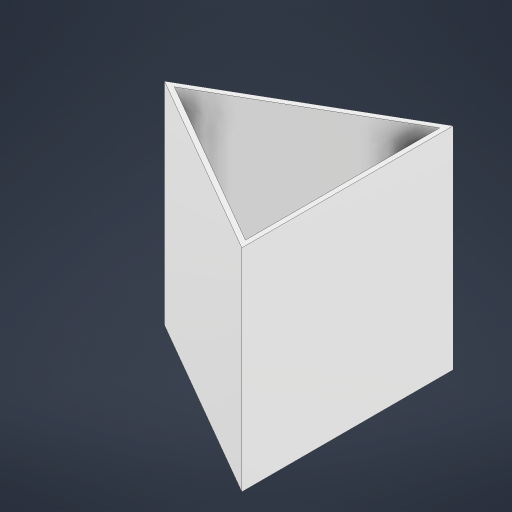
# Autodesk Inventor part: Triangle
Saved by Autodesk Inventor 2023 (Build 270158000, 158)
## iProperties
Created: 2023-11-15
Part Number: Triangle
Material: ABS Plastic
Document SubType Name: Modeling
Designer: dexter.hedman
Density: 1.06 g/cm^3
Appearance: Smooth - White
Author: dexter.hedman
Autodesk Inventor part; units mm, degrees
ref_plane "YZ Plane" through (0, 0, 0) normal (1, 0, 0) x (0, 1, 0)
ref_plane "XZ Plane" through (0, 0, 0) normal (0, 1, 0) x (-1, 0, 0)
ref_plane "XY Plane" through (0, 0, 0) normal (0, 0, 1) x (1, 0, 0)
sketch "Sketch2" plane through (0, 0, 0) normal (0, 1, 0) x (-1, 0, 0)
  line L0 (0, 27) -> (0, -27)
  line L1 (46.7654, 0) -> (0, -27)
  line L2 (46.7654, 0) -> (0, 27)
  line L3 (1.25, -24.8349) -> (1.25, 24.8349)
  line L4 (1.25, 24.8349) -> (44.2654, 0)
  line L5 (44.2654, 0) -> (1.25, -24.8349)
  point P0 (0, 0)
  dimension "d24" = 54
  dimension "d32" = 1.25
  constraints: 12 end point, 2 other
  measures "d24" distance of L0.end L0.start
  measures "d32" distance between parallel lines of L1 L5
extrude "Extrusion5" add sketch "Sketch2" along normal blind 54
body "Solid5"
